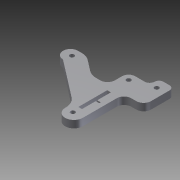
# Autodesk Inventor part: braket bawah
Saved by Autodesk Inventor 2012 (Build 160160000, 160)
## iProperties
Created: 2013-12-07
Part Number: braket bawah
Material: Default
Document SubType Name: Modeling
Designer: Irwan Haryanto
Density: 1 g/cm^3
Author: Irwan Haryanto
Autodesk Inventor part; units mm, degrees
ref_plane "YZ Plane" through (0, 0, 0) normal (1, 0, 0) x (0, 1, 0)
ref_plane "XZ Plane" through (0, 0, 0) normal (0, 1, 0) x (-1, 0, 0)
ref_plane "XY Plane" through (0, 0, 0) normal (0, 0, 1) x (1, 0, 0)
sketch "Sketch1" plane through (0, 0, 0) normal (0, 0, 1) x (1, 0, 0)
  line L0 (-3.96, 9.9) -> (-5, 9.9)
  line L1 (-3.96, 9.9) -> (-2.2612, 9.9)
  line L2 (-5, 9.9) -> (-2.2612, 9.9)
  arc A0 (3.8359, 7.8262) -> (-2.2612, 9.9) centre (-2.2612, -0.1) ccw
  arc A1 (3.8359, 7.8262) -> (-2.2612, 9.9) centre (-2.2612, -0.1) ccw
  line L3 (11.3141, 2.0738) -> (3.8359, 7.8262)
  line L4 (3.8359, 7.8262) -> (11.3141, 2.0738)
  line L5 (29.8, -3.5) -> (31.05, -3.5)
  line L6 (31.05, -23.3) -> (28.55, -23.3)
  line L7 (28.55, -23.3) -> (28.55, -3.5)
  line L8 (28.55, -23.3) -> (28.55, -3.5)
  line L9 (5.8588, -8.6221) -> (20.6471, -19.9978)
  line L10 (20.6471, -19.9978) -> (5.8588, -8.6221)
  line L11 (31.05, -12.9) -> (33.55, -12.9)
  line L12 (36.55, -13) -> (36.55, -5)
  line L13 (33.55, -13.9) -> (33.55, -12.9)
  line L14 (33.55, -12.9) -> (33.55, -13.9)
  line L15 (33.55, -12.9) -> (31.05, -12.9)
  line L16 (31.05, -13.9) -> (33.55, -13.9)
  line L17 (33.55, -13.9) -> (31.05, -13.9)
  line L18 (31.05, -23.3) -> (31.05, -13.9)
  line L19 (31.05, -13.9) -> (31.05, -23.3)
  line L20 (36.55, -5) -> (36.55, -28.3)
  line L21 (36.55, -13) -> (36.55, -14.9)
  line L22 (29.8, -23.3) -> (29.8, -28.3)
  line L23 (36.55, -14.9) -> (36.55, -28.3)
  line L24 (31.05, -12.9) -> (31.05, -3.5)
  line L25 (31.05, -3.5) -> (31.05, -12.9)
  arc A2 (29.8, 14.4) -> (25.3, 9.9) centre (29.8, 9.9) ccw
  arc A3 (29.8, 14.4) -> (25.3, 9.9) centre (29.8, 9.9) ccw
  arc A4 (36.3, 14.4) -> (39.7, 17.8) centre (36.3, 17.8) ccw
  arc A5 (36.3, 14.4) -> (39.7, 17.8) centre (36.3, 17.8) ccw
  line L26 (36.3, 14.4) -> (29.8, 14.4)
  line L27 (29.8, 14.4) -> (36.3, 14.4)
  line L28 (39.7, 17.8) -> (39.7, 17.8)
  arc A6 (-5, 9.9) -> (-10, 4.9) centre (-5, 4.9) ccw
  arc A7 (-5, 9.9) -> (-10, 4.9) centre (-5, 4.9) ccw
  arc A8 (-10, 4.7) -> (-5.7001, -0.2507) centre (-5, 4.7) ccw
  arc A9 (-10, 4.7) -> (-5.7001, -0.2507) centre (-5, 4.7) ccw
  line L29 (-10, 4.9) -> (-10, 4.7)
  line L30 (-10, 4.7) -> (-10, 4.9)
  line L31 (17.4112, 0) -> (20.3, 0)
  line L32 (28.55, -3.5) -> (29.8, -3.5)
  arc A10 (11.3141, 2.0738) -> (17.4112, 0) centre (17.4112, 10) ccw
  arc A11 (11.3141, 2.0738) -> (17.4112, 0) centre (17.4112, 10) ccw
  line L33 (50, 17.8) -> (50, 5)
  arc A12 (42.7, 20.8) -> (39.7, 17.8) centre (42.7, 17.8) ccw
  arc A13 (42.7, 20.8) -> (39.7, 17.8) centre (42.7, 17.8) ccw
  line L34 (44.7, 20.8) -> (42.7, 20.8)
  line L35 (42.7, 20.8) -> (46.7, 20.8)
  line L36 (44.7, 20.8) -> (47, 20.8)
  line L37 (50, 17.8) -> (50, 17.8)
  arc A14 (50, 17.8) -> (47, 20.8) centre (47, 17.8) ccw
  arc A15 (46.85, 20.7962) -> (46.7, 20.8) centre (46.7, 17.8) ccw
  line L38 (45, 0) -> (41.55, 0)
  arc A16 (41.55, 0) -> (36.55, -5) centre (41.55, -5) ccw
  arc A17 (45, 0) -> (50, 5) centre (45, 5) ccw
  line L39 (44.7, 0) -> (41.55, 0)
  line L40 (28.55, -3.5) -> (31.05, -3.5)
  arc A18 (41.55, 0) -> (36.55, -5) centre (41.55, -5) ccw
  arc A19 (44.7, 0) -> (44.85, 0.0023) centre (44.7, 5) ccw
  arc A20 (24.55, -28.3) -> (36.55, -28.3) centre (30.55, -28.3) ccw
  line L41 (31.05, -23.3) -> (28.55, -23.3)
  arc A21 (24.55, -27.924) -> (20.6471, -19.9978) centre (14.55, -27.924) ccw
  arc A22 (24.55, -27.924) -> (20.6471, -19.9978) centre (14.55, -27.924) ccw
  line L42 (24.55, -27.924) -> (24.55, -28.3)
  line L43 (24.55, -28.3) -> (24.55, -27.924)
  arc A23 (24.55, -28.3) -> (36.55, -28.3) centre (30.55, -28.3) ccw
  arc A24 (-4.2953, -0.8401) -> (-5.7001, -0.2507) centre (-6.1202, -3.2212) ccw
  arc A25 (-4.2953, -0.8401) -> (-5.7001, -0.2507) centre (-6.1202, -3.2212) ccw
  line L44 (5.8588, -8.6221) -> (-4.2953, -0.8401)
  line L45 (5.8588, -8.6221) -> (-4.2953, -0.8401)
  line L46 (25.3, 9.9) -> (25.3, 5)
  arc A26 (20.3, 0) -> (25.3, 5) centre (20.3, 5) ccw
  line L47 (25.3, 5) -> (25.3, 9.9)
  arc A27 (20.3, 0) -> (25.3, 5) centre (20.3, 5) ccw
  line L48 (17.4112, 0) -> (20.3, 0)
  point P0 (0, 0)
  point P1 (0, 0)
  dimension "d46" = 1.25
  dimension "d47" = 2.5
  dimension "d48" = 19.8
  dimension "d49" = 5
  dimension "d50" = 9.4
  dimension "d51" = 2.5
  dimension "d52" = 1
  dimension "d53" = 5
  dimension "d54" = 5
  dimension "d55" = 10
  dimension "d56" = 10
  dimension "d57" = 5
  dimension "d58" = 3
  dimension "d59" = 3
  dimension "d62" = 60
  dimension "d63" = 6.75
  dimension "d64" = 0.75
  dimension "d65" = 5.25
  dimension "d66" = 5
  constraints: 98 end point, 58 point on circle, 28 centre point, 21 tangent, 4 equal radius, 1 midpoint, 1 perpendicular, 1 point on line
  measures "d46" distance of L5.start L5.end
  measures "d47" distance of L6.start L6.end
  measures "d48" distance of L6.end L32.start
  measures "d49" distance of L22.start L22.end
  measures "d50" distance of L6.start L16.start
  measures "d51" distance of L16.start L13.start
  measures "d52" distance of L13.start L13.end
  measures "d53" radius of A16
  measures "d54" radius of A26
  measures "d55" radius of A21
  measures "d56" radius of A11
  measures "d57" radius of A6
  measures "d58" radius of A24
  measures "d59" radius of A12
  measures "d62" distance from line of L29.end L33
  measures "d63" distance from line of L20 L22.end
  measures "d64" distance of A20.centre L22.end
  measures "d65" distance from line of L42 L22.end
  measures "d66" distance from line of L22.end L6
extrude "Extrusion1" add sketch "Sketch1" along normal blind 5
sketch "Sketch2" plane through (0, 0, 5) normal (0, 0, 1) x (1, 0, 0)
  arc A0 (29.8, 14.4) -> (25.3, 9.9) centre (29.8, 9.9) ccw projected
  line L0 (17.4112, 0) -> (20.3, 0)
  circle A1 centre (44.04, 14.9) radius 1.5
  circle A2 centre (-3.96, 4.9) radius 1.5
  line L1 (29.8, -3.5) -> (31.05, -3.5)
  line L2 (31.05, -23.3) -> (28.55, -23.3)
  line L3 (28.55, -23.3) -> (28.55, -3.5)
  line L4 (28.55, -3.5) -> (29.8, -3.5)
  line L5 (29.8, -23.3) -> (29.8, -28.3)
  circle A3 centre (29.8, -28.3) radius 1.5
  line L6 (31.05, -23.3) -> (31.05, -13.9)
  line L7 (31.05, -13.9) -> (33.55, -13.9)
  line L8 (33.55, -13.9) -> (33.55, -12.9)
  line L9 (33.55, -12.9) -> (31.05, -12.9)
  line L10 (31.05, -12.9) -> (31.05, -3.5)
  line L11 (36.55, -14.9) -> (36.55, -28.3)
  line L12 (50, 17.8) -> (50, 5)
  line L13 (36.55, -13) -> (36.55, -14.9)
  arc A4 (24.55, -28.3) -> (36.55, -28.3) centre (30.55, -28.3) ccw
  line L14 (24.55, -27.924) -> (24.55, -28.3)
  line L15 (5.8588, -8.6221) -> (20.6471, -19.9978)
  circle A5 centre (29.8, 9.9) radius 1.5
  arc A6 (29.8, 14.4) -> (25.3, 9.9) centre (29.8, 9.9) ccw
  line L16 (25.3, 9.9) -> (25.3, 5)
  line L17 (36.55, -13) -> (36.55, -5)
  line L18 (45, 0) -> (41.55, 0)
  line L19 (36.3, 14.4) -> (29.8, 14.4)
  arc A7 (36.3, 14.4) -> (39.7, 17.8) centre (36.3, 17.8) ccw
  arc A8 (41.55, 0) -> (36.55, -5) centre (41.55, -5) ccw
  arc A9 (45, 0) -> (50, 5) centre (45, 5) ccw
  arc A10 (20.3, 0) -> (25.3, 5) centre (20.3, 5) ccw
  arc A11 (24.55, -27.924) -> (20.6471, -19.9978) centre (14.55, -27.924) ccw
  line L20 (-3.96, 9.9) -> (-2.2612, 9.9)
  line L21 (-3.96, 9.9) -> (-5, 9.9)
  line L22 (-10, 4.9) -> (-10, 4.7)
  line L23 (11.3141, 2.0738) -> (3.8359, 7.8262)
  arc A12 (11.3141, 2.0738) -> (17.4112, 0) centre (17.4112, 10) ccw
  arc A13 (3.8359, 7.8262) -> (-2.2612, 9.9) centre (-2.2612, -0.1) ccw
  arc A14 (-5, 9.9) -> (-10, 4.9) centre (-5, 4.9) ccw
  arc A15 (-10, 4.7) -> (-5.7001, -0.2507) centre (-5, 4.7) ccw
  line L24 (5.8588, -8.6221) -> (-4.2953, -0.8401)
  arc A16 (-4.2953, -0.8401) -> (-5.7001, -0.2507) centre (-6.1202, -3.2212) ccw
  line L25 (39.7, 17.8) -> (39.7, 17.8)
  line L26 (50, 17.8) -> (50, 17.8)
  line L27 (44.7, 20.8) -> (47, 20.8)
  line L28 (44.7, 20.8) -> (42.7, 20.8)
  arc A17 (42.7, 20.8) -> (39.7, 17.8) centre (42.7, 17.8) ccw
  arc A18 (50, 17.8) -> (47, 20.8) centre (47, 17.8) ccw
  line L29 (36.55, -5) -> (36.55, -28.3) projected
  point P0 (0, 0)
  dimension "d16" = 1.25
  dimension "d17" = 2.5
  dimension "d18" = 19.8
  dimension "d19" = 5
  dimension "d20" = 9.4
  dimension "d21" = 2.5
  dimension "d22" = 1
  dimension "d23" = 5
  dimension "d24" = 5
  dimension "d25" = 10
  dimension "d26" = 10
  dimension "d27" = 5
  dimension "d28" = 3
  dimension "d29" = 3
  dimension "d37" = 48
  dimension "d39" = 10
  dimension "d40" = 60
  dimension "d41" = 6.75
  dimension "d42" = 0.75
  dimension "d43" = 5.25
  dimension "d44" = 5
  dimension "d45" = 33.2
  constraints: 58 end point, 28 point on circle, 21 tangent, 18 centre point, 4 equal radius, 2 coincident, 1 midpoint, 1 perpendicular, 1 point on line
  measures "d16" distance of L1.start L1.end
  measures "d17" distance of L2.start L2.end
  measures "d18" distance of L2.end L3.end
  measures "d19" distance of L5.start L5.end
  measures "d20" distance of L2.start L6.end
  measures "d21" distance of L6.end L7.end
  measures "d22" distance of L7.end L8.end
  measures "d23" radius of A8
  measures "d24" radius of A10
  measures "d25" radius of A11
  measures "d26" radius of A12
  measures "d27" radius of A14
  measures "d28" radius of A16
  measures "d29" radius of A17
  measures "d37" horizontal distance of A1.centre A2.centre
  measures "d39" vertical distance of A1.centre A2.centre
  measures "d40" distance from line of L22.end L12
  measures "d41" distance from line of L29 L5.end
  measures "d42" distance of A4.centre L5.end
  measures "d43" distance from line of L14 L5.end
  measures "d44" distance from line of L5.end L2
  measures "d45" vertical distance of L5.end A2.centre
hole "Hole1" at (29.8, -28.3, 5) at (44.04, 14.9, 5) at (29.8, 9.9, 5) at (-3.96, 4.9, 5) direction (0, 0, -1) diameter 3 end through all
body "Solid1"
